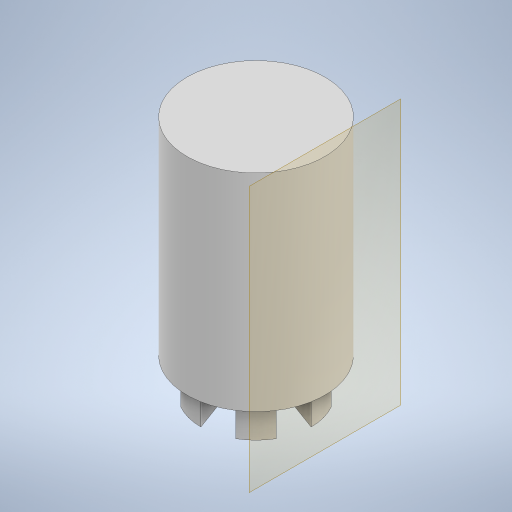
# Autodesk Inventor part: pot gövde
Saved by Autodesk Inventor 2023 (Build 270158000, 158)
## iProperties
Created: 2023-03-11
Part Number: pot gövde
Material: Generic
Document SubType Name: Modeling
Designer: Umut Yücesoy
Density: 1 g/cm^3
Appearance: Default
Author: Umut Yücesoy
Autodesk Inventor part; units mm, degrees
ref_plane "XZ Plane" through (0, 0, 0) normal (0, 1, 0) x (-1, 0, 0)
ref_plane "XY Plane" through (0, 0, 0) normal (0, 0, 1) x (1, 0, 0)
sketch "Sketch1" plane through (0, 0, 0) normal (0, 1, 0) x (-1, 0, 0)
  circle A0 centre (0, 0) radius 10
  dimension "d0" = 20
  constraints: 1 centre point, 1 coincident
  measures "d0" diameter of A0
extrude "Extrusion1" add sketch "Sketch1" along normal blind 30
sketch "Sketch2" plane through (0, 0, 0) normal (0, -1, 0) x (1, 0, 0)
  circle A0 centre (0, 0) radius 2.5
  dimension "d3" = 5
  constraints: 1 centre point, 1 coincident
  measures "d3" diameter of A0
extrude "Extrusion2" add sketch "Sketch2" along normal blind 5
sketch "Sketch3" plane through (0, -5, 0) normal (0, -1, 0) x (1, 0, 0)
  circle A0 centre (0, 0) radius 2.5 projected
  circle A1 centre (0, 0) radius 4.536
  circle A2 centre (0, 0) radius 8
  line L0 (0, -4.536) -> (0, -8)
  line L1 (0, 0) -> (4, -6.9282)
  line L2 (0, 0) -> (8, 0) construction
  point P0 (2.268, -3.9283)
  dimension "d6" = 9.072
  dimension "d7" = 16
  dimension "d8" = 60
  constraints: 6 end point, 2 coincident, 2 point on circle, 1 centre point, 1 equal length, 1 horizontal, 1 vertical, 3 other
  measures "d7" diameter of A2
  measures "d8" angle of L1 L2
extrude "Extrusion3" add sketch "Sketch3" against normal blind 5 contours A1 L1 A2 L0 picked at (1.6377, -6.621)
pattern_circular "Circular Pattern1" count 6 over 360 about axis through (0, 0, 0) along (0, -1, 0) of "Extrusion3"
ref_plane "Work Plane1" through (0, -5, 8) normal (1, 0, 0) x (0, 0, -1)
sketch "Sketch4" plane through (0, -5, 8) normal (1, 0, 0) x (0, 0, -1)
  line L0 (0, 0) -> (1.0718, 0) projected
  line L1 (0, 0) -> (3.4641, 2)
  line L2 (0, 0) -> (4, 0) construction
  line L3 (0, 0) -> (3.4641, 0)
  line L4 (3.4641, 2) -> (3.4641, 0)
  line L5 (5.732, 0) -> (5.732, 5) projected
  line L6 (8, -7) -> (8, 42) projected
  point P0 (8, 5)
  dimension "d15" = 4
  dimension "d16" = 30
  constraints: 8 end point, 1 equal length, 1 horizontal, 1 parallel, 1 point on line
  measures "d15" distance of L0.start L1.end
  measures "d16" angle of L2 L1
revolve "Revolution1" cut sketch "Sketch4" angle 360 about axis through (0, -10, 0) along (0, -1, 0)
ref_plane "Work Plane2" through (10, 0, 0) normal (1, 0, 0) x (0, 1, 0)
body "Solid1"
